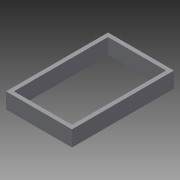
# Autodesk Inventor part: ChimeraLowTestFanNozzle
Saved by Autodesk Inventor 2015 SP1 (Build 190203100, 203)
## iProperties
Created: 2015-03-09
Part Number: ChimeraLowTestFanNozzle
Material: Generic
Document SubType Name: Modeling
Designer: Jack
Density: 1 g/cm^3
Appearance: Default
Author: Jack
Autodesk Inventor part; units mm, degrees
ref_plane "YZ Plane" through (0, 0, 0) normal (1, 0, 0) x (0, 1, 0)
ref_plane "XZ Plane" through (0, 0, 0) normal (0, 1, 0) x (-1, 0, 0)
ref_plane "XY Plane" through (0, 0, 0) normal (0, 0, 1) x (1, 0, 0)
sketch "Sketch1" plane through (0, 0, 0) normal (0, 0, 1) x (1, 0, 0)
  line L0 (0, 0) -> (16.8, 0)
  line L1 (16.8, 0) -> (16.8, 26)
  line L2 (16.8, 26) -> (0, 26)
  line L3 (0, 26) -> (0, 0)
  line L4 (15.8, 1) -> (1, 1)
  line L5 (1, 1) -> (1, 25)
  line L6 (1, 25) -> (15.8, 25)
  line L7 (15.8, 25) -> (15.8, 1)
  dimension "d0" = 16.8
  dimension "d1" = 26
  dimension "d2" = 1
  constraints: 16 end point, 4 parallel, 2 perpendicular, 1 horizontal, 3 other
  measures "d0" distance of L2.end L1.end
  measures "d1" distance of L1.end L0.end
  measures "d2" distance between parallel lines of L0 L4
extrude "Extrusion1" add sketch "Sketch1" along normal blind 8
body "Solid1"
